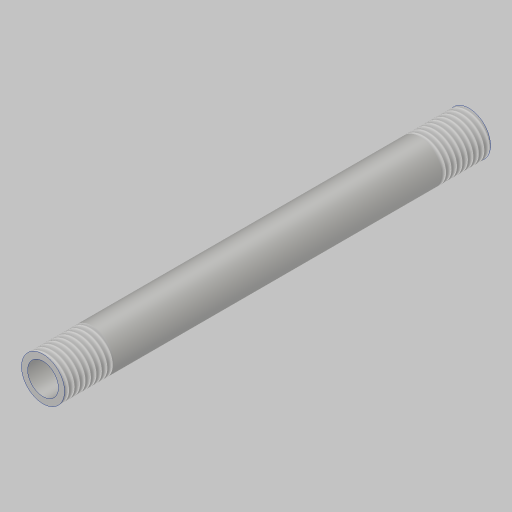
# Autodesk Inventor part: AR-006
Saved by Autodesk Inventor 2023.5 (Build 275446000, 446)
## iProperties
Created: 2025-01-11
Part Number: AR-006
Material: Aluminum 6061
Document SubType Name: Modeling
Designer: brand
Density: 2.7 g/cm^3
Appearance: Aluminum - Flat
Mass: 117.281 g
Surface Area: 277.422 cm^2
Volume: 43.4375 cm^3
Author: brand
Autodesk Inventor part; units mm, degrees
ref_plane "YZ Plane" through (0, 0, 0) normal (1, 0, 0) x (0, 1, 0)
ref_plane "XZ Plane" through (0, 0, 0) normal (0, 1, 0) x (-1, 0, 0)
ref_plane "XY Plane" through (0, 0, 0) normal (0, 0, 1) x (1, 0, 0)
sketch "Sketch1" plane through (0, 0, 0) normal (0, 0, 1) x (1, 0, 0)
  circle A0 centre (0, 0) radius 11.1125
  circle A1 centre (0, 0) radius 7.9375
  dimension "d0" = 22.225
  dimension "d1" = 3.175
  constraints: 2 centre point, 1 coincident
  measures "d0" diameter of A0
  measures "d1" radial gap between concentric circles of A0 A1
extrude "Extrusion1" add sketch "Sketch1" along normal mid plane 220.0402
thread "Thread1" size "7/8-9 UNC" class "2A" standard "ANSI Unified Screw Threads" length 25.4
thread "Thread2" size "7/8-9 UNC" class "2A" standard "ANSI Unified Screw Threads" length 25.4
equation "\"d6\" = d4"
equation "\"d4\" = 25.4"
body "Solid1"
